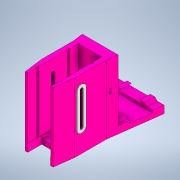
# Autodesk Inventor part: hull_main
Saved by Autodesk Inventor 2020 (Build 240168000, 168)
## iProperties
Created: 2019-09-18
Part Number: hull_main
Material: ABS Plastic
Document SubType Name: Modeling
Designer: suchanek
Density: 1.06 g/cm^3
Appearance: Smooth - White
Mass: 465.229 g
Surface Area: 1148.55 cm^2
Volume: 438.896 cm^3
Author: suchanek
Autodesk Inventor part; units mm, degrees
ref_plane "YZ Plane" through (0, 0, 0) normal (1, 0, 0) x (0, 1, 0)
ref_plane "XZ Plane" through (0, 0, 0) normal (0, 1, 0) x (-1, 0, 0)
ref_plane "XY Plane" through (0, 0, 0) normal (0, 0, 1) x (1, 0, 0)
sketch "Sketch1" plane through (0, 0, 0) normal (0, 1, 0) x (-1, 0, 0)
  line L0 (22.5, 50) -> (-22.5, 50)
  line L1 (-22.5, 50) -> (-22.5, 32)
  line L2 (-22.5, -50) -> (22.5, -50)
  line L3 (22.5, -50) -> (22.5, -32)
  line L4 (22.5, 50) -> (-22.5, -50) construction
  line L5 (-22.5, 50) -> (22.5, -50) construction
  line L6 (22.5, 50) -> (27.5, 50)
  line L7 (27.5, 50) -> (32.5, 12.0212)
  line L8 (45.6652, -150) -> (-45.6652, -150)
  line L9 (-27.5, 50) -> (-22.5, 50)
  line L10 (0, 0) -> (0, -26.257)
  line L11 (35.133, -70) -> (30.0899, -70)
  circle A0 centre (0, 22.5) radius 5.5
  line L12 (-5.5, 22.5) -> (-22.5, 22.5)
  line L13 (5.5, 22.5) -> (22.5, 22.5)
  line L14 (-32.5, 12.0212) -> (-32.5, -50)
  line L15 (-32.5, 12.0212) -> (-27.5, 50)
  line L16 (-32.5, -50) -> (-45.6652, -150)
  line L17 (32.5, 12.0212) -> (32.5, -50)
  line L18 (32.5, -50) -> (45.6652, -150)
  line L19 (22.5, 32) -> (24.5, 32)
  line L20 (24.5, 32) -> (24.5, 28)
  line L21 (24.5, 28) -> (22.5, 28)
  line L22 (22.5, 28) -> (22.5, 32)
  line L23 (0, 0) -> (10.1016, 0)
  line L24 (22.5, -32) -> (24.5, -32)
  line L25 (24.5, -32) -> (24.5, -28)
  line L26 (24.5, -28) -> (22.5, -28)
  line L27 (22.5, -28) -> (22.5, -32)
  line L28 (-22.5, 32) -> (-24.5, 32)
  line L29 (-24.5, 32) -> (-24.5, 28)
  line L30 (-24.5, 28) -> (-22.5, 28)
  line L31 (-22.5, 28) -> (-22.5, 32)
  line L32 (-24.5, -28) -> (-22.5, -28)
  line L33 (-22.5, -32) -> (-24.5, -32)
  line L34 (-24.5, -32) -> (-24.5, -28)
  line L35 (-22.5, -28) -> (-22.5, -32)
  line L36 (-22.5, 28) -> (-22.5, -28)
  line L37 (-22.5, 32) -> (-22.5, 28)
  line L38 (-22.5, -28) -> (-22.5, -32)
  line L39 (-22.5, -32) -> (-22.5, -50)
  line L40 (22.5, -28) -> (22.5, 28)
  line L41 (22.5, -32) -> (22.5, -28)
  line L42 (22.5, 28) -> (22.5, 32)
  line L43 (22.5, 32) -> (22.5, 50)
  line L44 (30.0899, -70) -> (28.1151, -55)
  line L45 (28.1151, -55) -> (0.5, -55)
  line L46 (-28.1151, -55) -> (-28.1151, -55)
  line L47 (-30.0899, -70) -> (-35.133, -70)
  line L48 (30.0899, -70) -> (-30.0899, -70)
  line L49 (-3.5, -55) -> (-28.1151, -55)
  line L50 (0.5, -55) -> (-3.5, -55)
  line L51 (-28.1151, -55) -> (-28.5101, -58)
  line L52 (-28.5101, -58) -> (-30.0899, -70)
  line L53 (-3.5, -55) -> (-0.5, -55)
  point P0 (-22.5, 0)
  point P1 (22.5, 0)
  dimension "d0" = 45
  dimension "d1" = 100
  dimension "d2" = 97.5
  dimension "d3" = 5
  dimension "d5" = 20
  dimension "d11" = 11
  dimension "d12" = 22.5
  dimension "d13" = 10
  dimension "d15" = 10
  dimension "d16" = 2
  dimension "d17" = 4
  dimension "d20" = 28
  dimension "d38" = 5
  dimension "d39" = 5
  dimension "d46" = 80
  constraints: 108 end point, 35 parallel, 15 point on line, 15 symmetric about line, 11 horizontal, 11 perpendicular, 3 vertical, 2 midpoint, 2 point on circle, 1 centre point, 1 collinear, 1 line through centre
  measures "d0" distance of L2.end L2.start
  measures "d1" distance of L2.start L0.end
  measures "d2" angle of L6 L7
  measures "d3" distance of L0.start L6.end
  measures "d5" distance between parallel lines of L11 L2
  measures "d11" diameter of A0
  measures "d12" distance of L10.start A0.centre
  measures "d13" distance between parallel lines of L1 L14
  measures "d15" distance between parallel lines of L3 L17
  measures "d16" distance of L20.end L21.end
  measures "d17" distance of L19.end L20.end
  measures "d20" distance between parallel lines of L23 L21
  measures "d38" distance between parallel lines of L2 L45
  measures "d39" distance between parallel lines of L16 L46
  measures "d46" distance between parallel lines of L8 L48
extrude "Extrusion1" add sketch "Sketch1" along normal blind 120 contours L6 L7 L17 L18 L11 L44 L45 L50 L49 L51 L52 L47 L16 L14 L15 L9 L1 L28 L29 L30 L36 L32 L34 L33 L39 L2 L3 L24 L25 L26 L40 L21 L20 L19 L43
extrude "Extrusion2" add sketch "Sketch1" against normal blind 15 contours L6 L7 L17 L18 L11 L44 L45 L50 L49 L51 L52 L47 L16 L14 L15 L9 L1 L28 L29 L30 L36 L32 L34 L33 L39 L2 L3 L24 L25 L26 L40 L21 L20 L19 L43 | L19 L20 L21 L22 | L31 L30 L29 L28 | L40 L27 L3 L2 L39 L35 L36 L12 A0 L13 | L18 L8 L16 L47 L48 L11 | L26 L25 L24 L27 | L35 L33 L34 L32 | L48 L52 L51 L49 L50 L45 L44
sketch "Sketch2" plane through (32.5, 120, 12.0212) normal (1, 0, 0) x (0, 0, -1)
  line L0 (12.0212, -90) -> (12.0212, -25) construction
  line L1 (15.0212, -90) -> (15.0212, -25)
  line L2 (9.0212, -25) -> (9.0212, -90)
  arc A0 (9.0212, -90) -> (15.0212, -90) centre (12.0212, -90) ccw
  arc A1 (15.0212, -25) -> (9.0212, -25) centre (12.0212, -25) ccw
  line L3 (0, 0) -> (62.0212, 0) projected
  point P0 (12.0212, -120)
  point P1 (12.0212, -57.5)
  dimension "d21" = 6
  dimension "d22" = 30
  dimension "d23" = 25
  constraints: 8 end point, 4 point on circle, 4 tangent, 2 centre point, 1 midpoint, 1 parallel, 1 point on line, 1 vertical
  measures "d21" diameter of A1
  measures "d22" distance of point (12.021, -120) L0.start
  measures "d23" distance from line of L3 L0.end
extrude "Extrusion3" cut sketch "Sketch2" against normal through all
sketch "Sketch3" plane through (32.5, 120, 12.0212) normal (1, 0, 0) x (0, 0, -1)
  line L0 (102.0212, -120) -> (142.0212, -120)
  line L1 (142.0212, -120) -> (142.0212, -125)
  line L2 (142.0212, -125) -> (102.0212, -125)
  line L3 (102.0212, -125) -> (102.0212, -120)
  line L4 (82.0212, -120) -> (162.0212, -120) projected
  line L5 (82.0212, -120) -> (82.0212, 0) projected
  point P0 (12.0212, -120)
  point P1 (82.0212, -120)
  dimension "d26" = 40
  dimension "d27" = 5
  dimension "d40" = 20
  constraints: 8 end point, 2 parallel, 1 collinear, 1 horizontal, 1 perpendicular
  measures "d26" distance of L1.end L2.end
  measures "d27" distance of L0.end L1.end
  measures "d40" distance from line of L5 L0.start
extrude "Extrusion4" cut sketch "Sketch3" along normal through all both and the other way through all
sketch "Sketch5" plane through (0, 0, 0) normal (0, 1, 0) x (1, 0, 0)
  line L0 (-30.0899, 70) -> (-35.133, 70) projected
  line L1 (37.7661, 90) -> (-37.7661, 90) projected
  line L2 (22.5, 70) -> (32.5, 70)
  line L3 (32.5, 70) -> (32.5, 90)
  line L4 (32.5, 90) -> (22.5, 90)
  line L5 (22.5, 90) -> (22.5, 70)
  line L6 (-43.0322, 130) -> (43.0322, 130) projected
  line L7 (-45.6652, 150) -> (45.6652, 150) projected
  line L8 (22.5, 130) -> (32.5, 130)
  line L9 (32.5, 130) -> (32.5, 150)
  line L10 (32.5, 150) -> (22.5, 150)
  line L11 (22.5, 150) -> (22.5, 130)
  line L12 (32.5, -12.0212) -> (32.5, 50) projected
  point P0 (0, 0)
  point P1 (35.133, 70)
  point P2 (32.5, 70)
  dimension "d32" = 10
  dimension "d33" = 0
  constraints: 16 end point, 6 point on line, 4 parallel, 2 horizontal, 2 perpendicular
  measures "d32" distance of L4.end L3.end
  measures "d33" distance between parallel lines of L12 L3
sketch "Sketch6" plane through (35.133, 120, -70) normal (0, 0, -1) x (-1, 0, 0)
  line L0 (12.633, -120) -> (17.633, -115)
  line L1 (12.633, -120) -> (19.7041, -120) construction
  line L2 (65.223, -120) -> (70.2661, -120) projected
  point P0 (35.133, -120)
  point P1 (12.633, -120)
  point P2 (0, -120)
  dimension "d34" = 45
  dimension "d35" = 5
  constraints: 4 end point, 1 equal length, 1 horizontal
  measures "d34" angle of L1 L0
  measures "d35" distance from line of L2 L0.end
sweep "Sweep1" add profiles "Sketch5" path "Sketch6" path curves L0
sketch "Sketch7" plane through (28.1151, 120, -55) normal (0, 0, -1) x (-1, 0, 0)
  line L0 (14.6151, -25) -> (24.6151, -25)
  line L1 (24.6151, -25) -> (24.6151, -95)
  line L2 (24.6151, -95) -> (14.6151, -95)
  line L3 (14.6151, -95) -> (14.6151, -25)
  line L4 (28.1151, -120) -> (28.1151, -109.7997)
  line L5 (0, 0) -> (56.2302, 0) projected
  line L6 (-17.5501, -120) -> (73.7804, -120) projected
  line L7 (5.6151, -120) -> (5.6151, 0) projected
  point P0 (28.6151, 0)
  dimension "d41" = 25
  dimension "d42" = 25
  dimension "d43" = 10
  dimension "d47" = 9
  constraints: 10 end point, 2 parallel, 1 horizontal, 1 perpendicular, 1 vertical
  measures "d41" distance between parallel lines of L5 L0
  measures "d42" distance between parallel lines of L6 L2
  measures "d43" distance between parallel lines of L1 L3
  measures "d47" distance between parallel lines of L7 L3
extrude "Extrusion5" cut sketch "Sketch7" against normal up to surface (5 mm away)
sketch "Sketch8" plane through (0, 0, 0) normal (0, 1, 0) x (1, 0, 0)
  arc A0 (5.5, -22.5) -> (-5.5, -22.5) centre (0, -22.5) ccw projected
  line L0 (-5.5, -22.5) -> (-22.5, -22.5) projected
  circle A1 centre (0, -22.5) radius 22.5
  point P0 (0, 0)
  constraints: 1 coincident, 1 horizontal alignment, 2 other
extrude "Extrusion6" cut sketch "Sketch8" against normal blind 5
sketch "Sketch9" plane through (0, 120, 0) normal (0, 1, 0) x (1, 0, 0)
  line L0 (35.133, 70) -> (30.0899, 70) projected
  line L1 (34.1244, 70) -> (31.623, 51)
  line L2 (31.623, 51) -> (-31.623, 51)
  line L3 (-31.623, 51) -> (-34.1244, 70)
  line L4 (-34.1244, 70) -> (34.1244, 70)
  line L5 (-35.133, 70) -> (-32.5, 50) projected
  line L6 (-22.5, 50) -> (22.5, 50) projected
  line L7 (32.5, 50) -> (35.133, 70) projected
  point P0 (0, 0)
  point P1 (31.4064, 80)
  point P2 (31.4064, 80)
  dimension "d57" = 1
  dimension "d58" = 1
  dimension "d59" = 1
  constraints: 8 end point, 3 parallel, 1 horizontal, 2 other
  measures "d57" distance between parallel lines of L7 L1
  measures "d58" distance between parallel lines of L6 L2
  measures "d59" distance between parallel lines of L5 L3
extrude "Extrusion7" add sketch "Sketch9" against normal blind 5
sketch "Sketch10" plane through (5.5, -15, 22.5) normal (0, 0, 1) x (1, 0, 0)
  circle A0 centre (8.5, 5) radius 2.2
  line L0 (-5.5, 15) -> (-5.5, 3.277)
  circle A1 centre (-19.5, 5) radius 2.2
  line L1 (0, 10) -> (0, 0) projected
  line L2 (17, 0) -> (0, 0) projected
  dimension "d65" = 8.5
  dimension "d66" = 5
  dimension "d67" = 4.4
  constraints: 2 centre point, 2 end point, 1 symmetric about line, 1 vertical, 1 other
  measures "d65" distance from line of L1 A0.centre
  measures "d66" distance from line of L2 A0.centre
  measures "d67" diameter of A0
extrude "Extrusion8" cut sketch "Sketch10" against normal blind 30
sketch "Sketch11" plane through (0, -15, 0) normal (0, -1, 0) x (1, 0, 0)
  line L0 (-18, 17.5) -> (-10, 17.5)
  line L1 (-10, 17.5) -> (-10, 13)
  line L2 (-10, 13) -> (-18, 13)
  line L3 (-18, 13) -> (-18, 17.5)
  arc A0 (-22.5, 22.5) -> (22.5, 22.5) centre (0, 22.5) ccw projected
  line L4 (0, 0) -> (0, 22.5)
  line L5 (18, 17.5) -> (10, 17.5)
  line L6 (10, 17.5) -> (10, 13)
  line L7 (10, 13) -> (18, 13)
  line L8 (18, 13) -> (18, 17.5)
  line L9 (-14, 17.5) -> (-14, 19.2413)
  line L10 (-5.5, 22.5) -> (-22.5, 22.5) projected
  dimension "d70" = 8
  dimension "d71" = 4.5
  dimension "d72" = 8.5
  dimension "d73" = 5
  constraints: 20 end point, 4 symmetric about line, 2 parallel, 2 vertical, 1 horizontal, 1 midpoint, 1 perpendicular
  measures "d70" distance of L0.start L0.end
  measures "d71" distance of L0.end L1.end
  measures "d72" distance from line of L10.end L9
  measures "d73" distance between parallel lines of L10 L0
extrude "Extrusion9" cut sketch "Sketch11" against normal blind 9
sketch "Sketch12" plane through (32.5, 120, 12.0212) normal (1, 0, 0) x (0, 0, -1)
  arc A0 (9.0212, -90) -> (15.0212, -90) centre (12.0212, -90) ccw projected
  line L0 (12.0212, -93) -> (12.0212, -22) construction
  arc A1 (15.0212, -25) -> (9.0212, -25) centre (12.0212, -25) ccw projected
  line L1 (15.0212, -90) -> (15.0212, -25)
  line L2 (9.0212, -25) -> (9.0212, -90)
  arc A2 (9.0212, -90) -> (15.0212, -90) centre (12.0212, -90) ccw
  arc A3 (15.0212, -25) -> (9.0212, -25) centre (12.0212, -25) ccw
  line L3 (12.0212, -90) -> (12.0212, -25) construction
  line L4 (21.0212, -90) -> (21.0212, -25)
  line L5 (3.0212, -25) -> (3.0212, -90)
  arc A4 (3.0212, -90) -> (21.0212, -90) centre (12.0212, -90) ccw
  arc A5 (21.0212, -25) -> (3.0212, -25) centre (12.0212, -25) ccw
  point P0 (12.0212, -120)
  point P1 (12.0212, -57.5)
  point P2 (12.0212, -57.5)
  dimension "d76" = 18
  constraints: 16 end point, 12 point on circle, 8 tangent, 4 centre point, 2 midpoint, 2 parallel, 2 point on line, 1 collinear, 1 vertical
  measures "d76" diameter of A5
extrude "Extrusion10" add sketch "Sketch12" along normal blind 1 separate body
mirror "Mirror1" about plane through (0, 0, 0) normal (1, 0, 0) of "Sweep1" bodies 1
mirror "Mirror2" about plane through (0, 0, 0) normal (1, 0, 0) of "Extrusion10" bodies 2
sketch "Sketch15" plane through (-28.1151, 0, -55) normal (0.9914449, 0, -0.1305262) x (-0.1305262, 0, -0.9914449)
  line L0 (15.1294, 0) -> (15.1294, 115) projected
  line L1 (0, 0) -> (0, 115) projected
  line L2 (15.1294, 60) -> (0, 60)
  line L3 (0, 60) -> (0, 69)
  line L4 (0, 69) -> (15.1294, 69)
  line L5 (15.1294, 69) -> (15.1294, 60)
  line L6 (0, 0) -> (15.1294, 0) projected
  line L7 (15.1294, 60) -> (25.1294, 60)
  line L8 (25.1294, 60) -> (25.1294, 69)
  line L9 (25.1294, 69) -> (15.1294, 69)
  line L10 (15.1294, 69) -> (15.1294, 60)
  point P0 (-58.1992, 0)
  point P1 (0, 60)
  dimension "d87" = 9
  dimension "d88" = 60
  dimension "d89" = 10
  constraints: 16 end point, 4 parallel, 2 horizontal, 2 perpendicular, 2 point on line, 1 collinear
  measures "d87" distance between parallel lines of L4 L2
  measures "d88" distance between parallel lines of L2 L6
  measures "d89" distance of L9.end L8.end
extrude "Extrusion13" cut sketch "Sketch15" against normal blind 3.5 contours L2 L1 L4 L0 | L0 L9 L8 L7 bodies 1
sketch "Sketch16" plane through (-31.5852, 0, -54.5432) normal (0.9914449, 0, -0.1305262) x (-0.1305262, 0, -0.9914449)
  line L0 (0, 60) -> (0, 69) projected
  line L1 (15.5902, 60) -> (0, 60) projected
  line L2 (0, 69) -> (3.5, 69)
  line L3 (3.5, 69) -> (3.5, 60)
  line L4 (3.5, 60) -> (0, 60)
  line L5 (0, 60) -> (0, 69)
  point P0 (-58.1992, 0)
  dimension "d92" = 3.5
  constraints: 8 end point, 2 parallel, 1 horizontal, 1 perpendicular, 1 point on line
  measures "d92" distance of L3.end L4.end
extrude "Extrusion14" cut sketch "Sketch16" against normal blind 5 bodies 1
mirror "Mirror4" about plane through (0, 0, 0) normal (1, 0, 0) of "Extrusion14", "Extrusion13" bodies 1
sketch "Sketch17" plane through (45.6652, 0, -150) normal (0, 0, -1) x (-1, 0, 0)
  line L0 (0, 0) -> (0, -15) projected
  line L1 (0, -0.4) -> (13.3309, -0.4)
  line L2 (13.3309, -0.4) -> (18.3309, 4.6)
  line L3 (18.3309, 4.6) -> (27.1996, 4.6)
  line L4 (27.1996, 4.6) -> (22.1996, -0.4)
  line L5 (22.1996, -0.4) -> (69.1309, -0.4)
  line L6 (69.1309, -0.4) -> (64.1309, 4.6)
  line L7 (64.1309, 4.6) -> (72.9996, 4.6)
  line L8 (72.9996, 4.6) -> (77.9996, -0.4)
  line L9 (77.9996, -0.4) -> (91.3305, -0.4)
  line L10 (91.3305, -0.4) -> (91.3305, 6)
  line L11 (91.3305, 6) -> (0, 6)
  line L12 (0, 6) -> (0, -0.4)
  line L13 (0, 0) -> (91.3305, 0) projected
  line L14 (13.1652, 0) -> (18.1652, 5) projected
  line L15 (18.1652, 5) -> (28.1652, 5) projected
  line L16 (23.1652, 0) -> (28.1652, 5) projected
  line L17 (68.1652, 0) -> (63.1652, 5) projected
  line L18 (78.1652, 0) -> (73.1652, 5) projected
  line L19 (91.3305, 0) -> (91.3305, -15) projected
  point P0 (45.6652, 0)
  dimension "d95" = 0.4
  dimension "d96" = 0.4
  dimension "d97" = 0.4
  dimension "d98" = 0.4
  dimension "d99" = 0.4
  dimension "d100" = 0.4
  dimension "d101" = 1
  constraints: 24 end point, 6 parallel, 6 point on line, 4 perpendicular, 1 horizontal
  measures "d95" distance between parallel lines of L13 L1
  measures "d96" distance between parallel lines of L14 L2
  measures "d97" distance between parallel lines of L15 L3
  measures "d98" distance between parallel lines of L16 L4
  measures "d99" distance between parallel lines of L17 L6
  measures "d100" distance between parallel lines of L18 L8
  measures "d101" distance between parallel lines of L11 L15
extrude "Extrusion15" cut sketch "Sketch17" against normal up to surface (80 mm away) contours L13 L2 L1 L0 | L12 L11 L10 L13 L8 L7 L6 L16 L15 L14 | L14 L15 L16 L13 L4 L3 L2 | L10 L9 L8 L13 | L13 L6 L5 L4 bodies 1
sketch "Sketch18" plane through (0, 120, 0) normal (0, 1, 0) x (1, 0, 0)
  line L0 (22.5, -50) -> (27.5, -50) projected
  line L1 (22.7, -50) -> (22.7, -32.2)
  line L2 (22.7, -32.2) -> (24.7, -32.2)
  line L3 (24.7, -32.2) -> (24.7, -27.8)
  line L4 (24.7, -27.8) -> (22.7, -27.8)
  line L5 (22.7, -27.8) -> (22.7, 27.8)
  line L6 (22.7, 27.8) -> (24.7, 27.8)
  line L7 (24.7, 27.8) -> (24.7, 32.2)
  line L8 (24.7, 32.2) -> (22.7, 32.2)
  line L9 (22.7, 32.2) -> (22.7, 50.2)
  line L10 (22.7, 50.2) -> (-22.7, 50.2)
  line L11 (28.1151, 55) -> (-28.1151, 55) projected
  line L12 (-22.7, 50.2) -> (-22.7, 32.2)
  line L13 (-22.7, 32.2) -> (-24.7, 32.2)
  line L14 (-24.7, 32.2) -> (-24.7, 27.8)
  line L15 (-24.7, 27.8) -> (-22.7, 27.8)
  line L16 (-22.7, 27.8) -> (-22.7, -27.8)
  line L17 (-22.7, -27.8) -> (-24.7, -27.8)
  line L18 (-24.7, -27.8) -> (-24.7, -32.2)
  line L19 (-24.7, -32.2) -> (-22.7, -32.2)
  line L20 (-22.7, -32.2) -> (-22.7, -50)
  line L21 (-22.7, -50) -> (22.7, -50)
  line L22 (22.5, -32) -> (22.5, -50) projected
  line L23 (24.5, -32) -> (22.5, -32) projected
  line L24 (24.5, -28) -> (24.5, -32) projected
  line L25 (22.5, -28) -> (24.5, -28) projected
  line L26 (22.5, 32) -> (24.5, 32) projected
  line L27 (24.5, 28) -> (22.5, 28) projected
  line L28 (-22.5, 50) -> (22.5, 50) projected
  line L29 (-22.5, 32) -> (-22.5, 50) projected
  line L30 (-24.5, 28) -> (-24.5, 32) projected
  line L31 (-22.5, 28) -> (-24.5, 28) projected
  line L32 (-22.5, -50) -> (-22.5, -32) projected
  line L33 (-24.5, -28) -> (-22.5, -28) projected
  point P0 (0, 0)
  dimension "d104" = 0.2
  dimension "d105" = 0.2
  dimension "d106" = 0.2
  dimension "d107" = 0.2
  dimension "d108" = 0.2
  dimension "d109" = 0.2
  dimension "d110" = 0.2
  dimension "d111" = 0.2
  dimension "d112" = 0.2
  dimension "d113" = 0.2
  dimension "d114" = 0.2
  dimension "d115" = 0.2
  constraints: 40 end point, 14 point on line, 11 perpendicular, 1 horizontal, 1 parallel, 1 vertical
  measures "d104" distance between parallel lines of L22 L1
  measures "d105" distance between parallel lines of L23 L2
  measures "d106" distance between parallel lines of L24 L3
  measures "d107" distance between parallel lines of L4 L25
  measures "d108" distance between parallel lines of L26 L8
  measures "d109" distance between parallel lines of L27 L6
  measures "d110" distance between parallel lines of L28 L10
  measures "d111" distance between parallel lines of L29 L12
  measures "d112" distance between parallel lines of L30 L14
  measures "d113" distance between parallel lines of L31 L15
  measures "d114" distance between parallel lines of L32 L20
  measures "d115" distance between parallel lines of L33 L17
extrude "Extrusion16" cut sketch "Sketch18" against normal up to surface (120 mm away) bodies 1
sketch "Sketch19" plane through (0, 0, 0) normal (0, 1, 0) x (1, 0, 0)
  line L0 (35.133, 70) -> (-35.133, 70) projected
  line L1 (-30.2916, 70) -> (-28.2905, 54.8)
  line L2 (-28.2905, 54.8) -> (28.2905, 54.8)
  line L3 (28.2905, 54.8) -> (30.2916, 70)
  line L4 (30.0899, 70) -> (28.1151, 55) projected
  line L5 (-28.1151, 55) -> (-30.0899, 70) projected
  line L6 (-28.1151, 55) -> (28.1151, 55) projected
  point P0 (0, 0)
  dimension "d118" = 0.2
  dimension "d119" = 0.2
  dimension "d120" = 0.2
  constraints: 6 end point, 3 parallel, 2 point on line
  measures "d118" distance between parallel lines of L5 L1
  measures "d119" distance between parallel lines of L6 L2
  measures "d120" distance between parallel lines of L4 L3
extrude "Extrusion17" cut sketch "Sketch19" along normal blind 116 and the other way blind 0.4 bodies 1
chamfer "Chamfer1" distance 2 angle 45 1 edges at (0, 116, -70)
fillet "Fillet1" radius 6 1 edges at (0, 116, -68)
fillet "Fillet2" radius 2 2 edges at (-32.044, 64.5, -58.013) (32.044, 64.5, -58.013)
equation "\"d96\" = d95"
equation "\"d97\" = d95"
equation "\"d98\" = d95"
equation "\"d99\" = d95"
equation "\"d100\" = d95"
equation "\"d105\" = d104"
equation "\"d106\" = d104"
equation "\"d107\" = d104"
equation "\"d108\" = d104"
equation "\"d109\" = d104"
equation "\"d110\" = d104"
equation "\"d111\" = d104"
equation "\"d112\" = d104"
equation "\"d113\" = d104"
equation "\"d114\" = d104"
equation "\"d115\" = d104"
equation "\"d119\" = d118"
equation "\"d120\" = d118"
body "Solid1"
body "Solid3"
